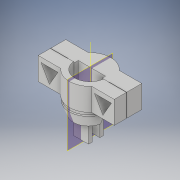
# Autodesk Inventor part: ECoG_holder_4p0
Saved by Autodesk Inventor 2017 (Build 210142000, 142)
## iProperties
Created: 2016-11-02
Part Number: ECoG_holder_4p0
Material: Generic
Document SubType Name: Modeling
Designer: Camilo
Density: 1 g/cm^3
Appearance: Default
Author: Camilo
Autodesk Inventor part; units mm, degrees
ref_plane "YZ Plane" through (0, 0, 0) normal (1, 0, 0) x (0, 1, 0)
ref_plane "XZ Plane" through (0, 0, 0) normal (0, 1, 0) x (-1, 0, 0)
ref_plane "XY Plane" through (0, 0, 0) normal (0, 0, 1) x (1, 0, 0)
sketch "Sketch1" plane through (0, 0, 0) normal (0, 0, 1) x (1, 0, 0)
  line L0 (0, 0) -> (0, -7.0002) construction
  line L1 (0, -7.0002) -> (0.78, -7.0002) construction
  line L2 (0.78, 0) -> (0.78, -7.0002) construction
  line L3 (0, 0) -> (0.78, 0) construction
  line L4 (0.39, -7.0002) -> (0.39, 0) construction
  circle A0 centre (0.39, -3.5001) radius 5.5
  dimension "d0" = 11
  constraints: 3 midpoint, 2 end point, 1 centre point
  measures "d0" diameter of A0
extrude "Extrusion1" add sketch "Sketch1" against normal blind 4.5 and the other way blind 1.5
shell "Shell1" thickness 1.5 removed faces 1 at (2.1701, -3.9389, -4.5)
sketch "Sketch2" plane through (0.39, -3.5001, 0) normal (0, 0, -1) x (-1, 0, 0)
  line L0 (0.39, 3.5001) -> (0.39, -3.5001) construction
  line L1 (0.39, -3.5001) -> (-0.39, -3.5001) construction
  line L2 (-0.39, 3.5001) -> (-0.39, -3.5001) construction
  line L3 (0.39, 3.5001) -> (-0.39, 3.5001) construction
  circle A0 centre (0, 0) radius 4 construction
  line L4 (0.515, -3.6251) -> (0.515, 3.6251)
  line L5 (0.515, 3.6251) -> (-0.515, 3.6251)
  line L6 (-0.515, 3.6251) -> (-0.515, -3.6251)
  line L7 (-0.515, -3.6251) -> (0.515, -3.6251)
  line L8 (-0.39, -3.6251) -> (-0.39, -3.9809)
  line L9 (-0.39, 3.6251) -> (-0.39, 3.9809)
  arc A1 (-0.39, -3.9809) -> (-0.39, 3.9809) centre (0, 0) ccw
  dimension "d6" = 0.125
  constraints: 12 end point, 4 point on circle, 4 point on line, 1 centre point, 1 vertical, 3 other
  measures "d6" distance between parallel lines of L0 L4
extrude "Extrusion2" add sketch "Sketch2" along normal up to surface (4.5 mm away) contours L4 L5 L9 A1 L8 L7
sketch "Sketch3" plane through (0.39, -3.5001, -4.5) normal (0, 0, -1) x (-1, 0, 0)
  arc A0 (-0.39, 3.9809) -> (-0.39, -3.9809) centre (0, 0) ccw construction
  line L0 (-0.39, 3.9809) -> (-0.39, 3.6251) construction
  line L1 (-0.39, 3.6251) -> (0.515, 3.6251) construction
  line L2 (0.515, 3.6251) -> (0.515, -3.6251) construction
  line L3 (0.515, -3.6251) -> (-0.39, -3.6251) construction
  line L4 (-0.39, -3.6251) -> (-0.39, -3.9809) construction
  circle A1 centre (0, 0) radius 5.5 construction
  circle A2 centre (0, 0) radius 5.5 projected
  line L5 (-0.39, -5.4862) -> (-0.39, 5.4862)
  point P0 (0.39, 3.5001)
  constraints: 4 point on circle, 2 end point, 1 point on line, 1 vertical
split body "Split1" sketch "Sketch3" result two bodies curves L5 first body at (4.651, -4.9471, -3)
sketch "Sketch11" plane through (0, 0, -4.5) normal (0, 0, -1) x (-1, 0, 0)
  line L0 (-0.78, 1.986) -> (-0.78, 0.125) construction
  line L1 (-0.78, 0.125) -> (0.125, 0.125) construction
  line L2 (0.125, 0.125) -> (0.125, -7.1252) construction
  line L3 (0.125, -7.1252) -> (-0.78, -7.1252) construction
  line L4 (-0.78, -7.1252) -> (-0.78, -8.9863) construction
  arc A0 (-0.78, -8.9863) -> (-0.78, 1.986) centre (-0.39, -3.5001) ccw construction
  arc A1 (-0.78, -8.9863) -> (-0.78, 1.986) centre (-0.39, -3.5001) ccw construction
  line L5 (-0.73, -13.6055) -> (3.27, -13.6055)
  line L6 (3.27, -13.6055) -> (3.27, -7.6055)
  line L7 (3.27, -7.6055) -> (-0.73, -7.6055)
  line L8 (-0.73, -7.6055) -> (-0.73, -13.6055)
  line L9 (-0.39, -3.5001) -> (5.11, -3.5001) construction
  line L10 (0.125, 0.125) -> (-0.78, 0.125) construction
  line L11 (-0.78, 0.125) -> (-0.78, 1.986) construction
  line L12 (-0.73, 6.6053) -> (3.27, 6.6053)
  line L13 (3.27, 6.6053) -> (3.27, 0.6053)
  line L14 (3.27, 0.6053) -> (-0.73, 0.6053)
  line L15 (-0.73, 0.6053) -> (-0.73, 6.6053)
  point P0 (0, 0)
  dimension "d38" = 0.05
  dimension "d39" = 4
  dimension "d40" = 6
  constraints: 22 end point, 4 symmetric about line, 3 point on circle, 2 parallel, 1 horizontal, 1 perpendicular
  measures "d38" distance between parallel lines of L8 L4
  measures "d39" distance of L5.start L5.end
  measures "d40" distance of L5.end L6.end
extrude "Extrusion10" add sketch "Sketch11" against normal up to surface (6 mm away) bodies 3
sketch "Sketch12" plane through (0, 0, -4.5) normal (0, 0, -1) x (-1, 0, 0)
  line L0 (-0.78, 1.986) -> (-0.78, 0.4808) construction
  arc A0 (-0.78, 1.986) -> (-5.89, -3.5001) centre (-0.39, -3.5001) ccw construction
  arc A1 (-5.89, -3.5001) -> (-0.78, -8.9863) centre (-0.39, -3.5001) ccw construction
  line L1 (-0.78, -7.4811) -> (-0.78, -8.9863) construction
  arc A2 (-0.78, 0.4808) -> (-0.78, -7.4811) centre (-0.39, -3.5001) ccw construction
  line L2 (-0.39, -3.5001) -> (-5.89, -3.5001) construction
  arc A3 (-0.78, 1.986) -> (-5.89, -3.5001) centre (-0.39, -3.5001) ccw projected
  line L3 (-0.83, 6.6053) -> (-4.05, 6.6053)
  line L4 (-4.05, 6.6053) -> (-4.05, 0.6053)
  line L5 (-4.05, 0.6053) -> (-0.83, 0.6053)
  line L6 (-0.83, 0.6053) -> (-0.83, 6.6053)
  line L7 (-0.73, 6.6053) -> (3.27, 6.6053) projected
  line L8 (-0.78, -8.9863) -> (-0.78, -7.4811) construction
  line L9 (-0.83, -13.6055) -> (-4.05, -13.6055)
  line L10 (-4.05, -13.6055) -> (-4.05, -7.6055)
  line L11 (-4.05, -7.6055) -> (-0.83, -7.6055)
  line L12 (-0.83, -7.6055) -> (-0.83, -13.6055)
  point P0 (0, 0)
  dimension "d43" = 0.05
  dimension "d44" = 6
  dimension "d46" = 0
  constraints: 20 end point, 4 symmetric about line, 2 horizontal, 2 parallel, 2 point on circle, 1 perpendicular
  measures "d43" distance between parallel lines of L6 L0
  measures "d44" distance of L3.end L4.end
  measures "d46" distance between parallel lines of L3 L7
extrude "Extrusion11" add sketch "Sketch12" against normal up to surface (6 mm away) bodies 2
sketch "Sketch13" plane through (0.73, 1.9894, -4.5) normal (1, 0, 0) x (0, 0, -1)
  line L0 (0, 0) -> (-6, 0) construction
  line L1 (0, 0) -> (0, 4.6159) construction
  line L2 (0, 4.6159) -> (-6, 4.6159) construction
  line L3 (-6, 4.6159) -> (-6, 0) construction
  line L4 (-6, -10.979) -> (0, -10.979) construction
  line L5 (-6, -10.979) -> (-6, -15.5949) construction
  line L6 (0, -15.5949) -> (-6, -15.5949) construction
  line L7 (0, -10.979) -> (0, -15.5949) construction
  line L8 (0, -1.8644) -> (0, -9.1146) construction
  line L9 (-4.5, -1.8644) -> (0, -1.8644) construction
  line L10 (-4.5, -9.1146) -> (-4.5, -1.8644) construction
  line L11 (-4.5, -9.1146) -> (0, -9.1146) construction
  line L12 (0, -10.9756) -> (-6, -10.9756) construction
  line L13 (0, -15.5949) -> (0, -9.5949) construction
  line L14 (-5.15, 1.6159) -> (-1.25, 3.8676)
  line L15 (-1.25, 3.8676) -> (-1.25, -0.6357)
  line L16 (-1.25, -0.6357) -> (-5.15, 1.6159)
  line L17 (-5.15, -12.5949) -> (-1.25, -10.3432)
  line L18 (-1.25, -10.3432) -> (-1.25, -14.8466)
  line L19 (-1.25, -14.8466) -> (-5.15, -12.5949)
  circle A0 centre (-2.55, 1.6159) radius 1.3
  point P0 (-4.5, -1.9894)
  point P1 (-2.55, -12.5949)
  dimension "d77" = 2.6
  dimension "d78" = 1.25
  dimension "d79" = 3
  dimension "d80" = 3
  constraints: 12 end point, 2 collinear, 2 vertical, 1 centre point, 1 coincident, 1 tangent, 14 other
  measures "d77" diameter of A0
  measures "d78" distance between parallel lines of L1 L15
  measures "d79" distance from line of point (-2.55, 1.616) L2
  measures "d80" distance from line of point (-2.55, -12.595) L6
extrude "Extrusion12" cut sketch "Sketch13" against normal blind 2.5 and the other way blind 0.2 bodies 3
sketch "Sketch14" plane through (0.83, 1.9823, -4.5) normal (-1, 0, 0) x (0, 0, 1)
  line L0 (1.25, 3.8747) -> (1.25, -0.6286) construction
  line L1 (5.15, 1.623) -> (1.25, 3.8747) construction
  line L2 (1.25, -0.6286) -> (5.15, 1.623) construction
  line L3 (5.15, -12.5878) -> (1.25, -10.3361) construction
  line L4 (1.25, -10.3361) -> (1.25, -14.8394) construction
  line L5 (1.25, -14.8394) -> (5.15, -12.5878) construction
  line L6 (1.25, 3.8747) -> (1.25, -0.6286)
  line L7 (1.25, -0.6286) -> (5.15, 1.623)
  line L8 (5.15, 1.623) -> (1.25, 3.8747)
  line L9 (1.25, -10.3361) -> (5.15, -12.5878)
  line L10 (5.15, -12.5878) -> (1.25, -14.8394)
  line L11 (1.25, -14.8394) -> (1.25, -10.3361)
  point P0 (4.5, -1.9823)
  dimension "d52" = 0
  constraints: 12 end point, 1 collinear, 4 other
  measures "d52" distance between parallel lines of L1 L8
extrude "Extrusion13" cut sketch "Sketch14" against normal through all bodies 2
sketch "Sketch15" plane through (0, 0, 1.5) normal (0, 0, 1) x (1, 0, 0)
  arc A0 (0.73, -8.9896) -> (0.78, -8.9863) centre (0.39, -3.5001) ccw construction
  line L0 (0.78, -8.9863) -> (0.78, 1.986) construction
  arc A1 (0.78, 1.986) -> (0.73, 1.9894) centre (0.39, -3.5001) ccw construction
  line L1 (0.73, 6.6053) -> (0.73, 1.9894) construction
  line L2 (-3.27, 6.6053) -> (0.73, 6.6053) construction
  line L3 (-3.27, 0.6053) -> (-3.27, 6.6053) construction
  arc A2 (-3.27, 0.6053) -> (-3.27, -7.6055) centre (0.39, -3.5001) ccw construction
  line L4 (-3.27, -13.6055) -> (-3.27, -7.6055) construction
  line L5 (0.73, -13.6055) -> (-3.27, -13.6055) construction
  line L6 (0.73, -8.9896) -> (0.73, -13.6055) construction
  line L7 (0.78, -1.0001) -> (-0.22, -1.0001)
  line L8 (-0.22, -1.0001) -> (-0.22, -6.0001)
  line L9 (-0.22, -6.0001) -> (0.78, -6.0001)
  line L10 (0.78, -6.0001) -> (0.78, -1.0001)
  line L11 (0.78, -0.0001) -> (-1.22, -0.0001)
  line L12 (-1.22, -0.0001) -> (-1.22, -7.0001)
  line L13 (-1.22, -7.0001) -> (0.78, -7.0001)
  line L14 (0.78, -7.0001) -> (0.78, -0.0001)
  line L15 (0.78, -8.9863) -> (0.78, 1.986) projected
  point P0 (0, 0)
  point P1 (0.78, -3.5001)
  point P2 (0.78, -3.5001)
  dimension "d55" = 5
  dimension "d56" = 1
  dimension "d57" = 1
  dimension "d58" = 1
  constraints: 16 end point, 4 midpoint, 4 parallel, 2 horizontal, 2 perpendicular
  measures "d55" distance of L7.end L8.end
  measures "d56" distance of L8.end L9.end
  measures "d57" distance between parallel lines of L12 L8
  measures "d58" distance between parallel lines of L9 L13
extrude "Extrusion14" add sketch "Sketch15" along normal blind 2 contours L7 L8 L9 L14 L13 L12 L11 bodies 3
sketch "Sketch16" plane through (0, 0, 1.5) normal (0, 0, 1) x (1, 0, 0)
  arc A0 (0.83, 1.9823) -> (0.78, 1.986) centre (0.39, -3.5001) ccw construction
  line L0 (0.78, -8.9863) -> (0.78, 1.986) construction
  arc A1 (0.78, -8.9863) -> (0.83, -8.9825) centre (0.39, -3.5001) ccw construction
  line L1 (0.83, -13.6055) -> (0.83, -8.9825) construction
  line L2 (4.05, -13.6055) -> (0.83, -13.6055) construction
  line L3 (4.05, -7.6055) -> (4.05, -13.6055) construction
  arc A2 (4.05, -7.6055) -> (4.05, 0.6053) centre (0.39, -3.5001) ccw construction
  line L4 (4.05, 6.6053) -> (4.05, 0.6053) construction
  line L5 (0.83, 6.6053) -> (4.05, 6.6053) construction
  line L6 (0.83, 1.9823) -> (0.83, 6.6053) construction
  line L7 (-0.22, -1.0001) -> (0.78, -1.0001) construction
  line L8 (0.78, -1.0001) -> (0.78, -0.0001) projected
  line L9 (0.78, -0.0001) -> (-1.22, -0.0001) construction
  line L10 (-1.22, -0.0001) -> (-1.22, -7.0001) construction
  line L11 (-1.22, -7.0001) -> (0.78, -7.0001) construction
  line L12 (0.78, -7.0001) -> (0.78, -6.0001) projected
  line L13 (0.78, -6.0001) -> (-0.22, -6.0001) construction
  line L14 (-0.22, -6.0001) -> (-0.22, -1.0001) construction
  line L15 (1.78, -1.0001) -> (0.78, -1.0001)
  line L16 (0.78, -0.0001) -> (2.78, -0.0001)
  line L17 (2.78, -0.0001) -> (2.78, -7.0001)
  line L18 (2.78, -7.0001) -> (0.78, -7.0001)
  line L19 (0.78, -6.0001) -> (1.78, -6.0001)
  line L20 (1.78, -6.0001) -> (1.78, -1.0001)
  point P0 (0, 0)
  point P1 (1.56, 0)
  point P2 (1.17, -3.5001)
  point P3 (1.17, -3.5001)
  point P4 (1.17, -3.5001)
  constraints: 12 end point, 8 symmetric about line
extrude "Extrusion15" add sketch "Sketch16" along normal blind 2 bodies 2
sketch "Sketch17" plane through (0.78, -7.1252, 0) normal (1, 0, 0) x (0, 0, -1)
  line L0 (-1.5, 9.1113) -> (4.5, 9.1113) projected
  line L1 (-1.5, 9.1113) -> (-1.5, 7.1113)
  line L2 (-1.5, 9.1113) -> (0.5, 9.1113) construction
  line L3 (-1.5, 7.1251) -> (-1.5, 9.1113) projected
  line L4 (-1.5, 7.1251) -> (-5.5, 7.1251)
  line L5 (-5.5, 7.1251) -> (-5.5, 7.6251)
  line L6 (-5.5, 7.6251) -> (-1.5, 9.1113)
  line L7 (-7.5, 3.6251) -> (6.5, 3.6251) projected
  line L8 (-2, 8.9255) -> (-1.5, 8.9255) construction
  line L9 (-1.5, 8.9255) -> (-1.5, 8.6255)
  line L10 (-1.5, 8.6255) -> (-2, 8.6255)
  line L11 (-2, 8.6255) -> (-2, 8.9255)
  point P0 (0, 7.1252)
  dimension "d63" = 2
  dimension "d64" = 90
  dimension "d65" = 4
  dimension "d66" = 0.5
  dimension "d69" = 0.5
  dimension "d70" = 0.3
  constraints: 18 end point, 3 horizontal, 3 perpendicular, 2 parallel, 2 point on line, 1 vertical
  measures "d63" distance of L0.start L1.end
  measures "d64" angle of L1 L2
  measures "d65" distance of L3.start L4.end
  measures "d66" distance of L4.end L5.end
  measures "d69" distance of L9.end L10.end
  measures "d70" distance of L10.end L8.start
revolve "Revolution1" add sketch "Sketch17" angle 180 about axis through (0.78, -3.5001, 0) along (0, 0, 1) bodies 3
sketch "Sketch18" plane through (0.78, -7.1252, 0) normal (-1, 0, 0) x (0, 0, 1)
  line L0 (-2.1546, -1.861) -> (1.5, -1.861) construction
  line L1 (-4.5, 0) -> (-4.5, -1.861) construction
  line L2 (0, 0) -> (-4.5, 0) construction
  line L3 (0, 7.2502) -> (0, 0) construction
  line L4 (0, 7.2502) -> (-4.5, 7.2502) construction
  line L5 (-4.5, 9.1113) -> (-4.5, 7.2502) construction
  line L6 (1.5, 9.1113) -> (-2.1546, 9.1113) construction
  line L7 (5.5, 7.6251) -> (1.5, 9.1113) construction
  line L8 (5.5, 7.1251) -> (5.5, 7.6251) construction
  line L9 (3.5, 7.1251) -> (5.5, 7.1251) construction
  line L10 (3.5, 6.1251) -> (3.5, 7.1251) construction
  line L11 (3.5, 6.1251) -> (1.5, 6.1251) construction
  line L12 (1.5, 1.1251) -> (1.5, 6.1251) construction
  line L13 (1.5, 1.1251) -> (3.5, 1.1251) construction
  line L14 (3.5, 0.1251) -> (3.5, 1.1251) construction
  line L15 (3.5, 0.1251) -> (5.5, 0.1251) construction
  line L16 (5.5, 0.1251) -> (5.5, -0.3749) construction
  line L17 (5.5, -0.3749) -> (1.5, -1.861) construction
  line L18 (5.5, 7.6251) -> (1.5, 9.1113) projected
  line L19 (1.5, 7.1251) -> (3.5, 7.1251) projected
  line L20 (1.5, 9.1113) -> (1.5, 7.1251)
  line L21 (1.5, 7.1251) -> (5.5, 7.1251)
  line L22 (1.5, 9.1113) -> (1.5, -1.861) projected
  line L23 (5.5, 7.6251) -> (1.5, 9.1113)
  line L24 (5.5, 7.1251) -> (5.5, 7.6251) projected
  line L25 (5.5, 7.1251) -> (5.5, 7.6251)
  line L26 (7.5, 3.6251) -> (-6.5, 3.6251) projected
  line L27 (-3.25, 8.4789) -> (-2.1546, 9.1113) projected
  line L28 (-2.1546, -1.861) -> (-3.25, -1.2286) projected
  line L29 (-3.25, -1.2286) -> (-3.25, -1.861) projected
  line L30 (-4.5, -1.861) -> (-3.25, -1.861) projected
  line L31 (-3.25, 9.1113) -> (-4.5, 9.1113) projected
  line L32 (-3.25, 9.1113) -> (-3.25, 8.4789) projected
  point P0 (0, 7.1252)
  constraints: 8 end point, 2 collinear, 2 perpendicular
revolve "Revolution2" add sketch "Sketch18" angle 180 about axis through (0.78, -3.5001, 0) along (0, 0, -1) bodies 2
sketch "Sketch19" plane through (0.78, -7.1252, 0) normal (1, 0, 0) x (0, 0, -1)
  line L0 (2.1546, -1.861) -> (-1.5, -1.861) construction
  line L1 (4.5, 0) -> (4.5, -1.861) construction
  line L2 (0, 0) -> (4.5, 0) construction
  line L3 (0, 7.2502) -> (0, 0) construction
  line L4 (0, 7.2502) -> (4.5, 7.2502) construction
  line L5 (4.5, 9.1113) -> (4.5, 7.2502) construction
  line L6 (-1.5, 9.1113) -> (2.1546, 9.1113) construction
  line L7 (-5.5, 7.6251) -> (-1.5, 9.1113) construction
  line L8 (-5.5, 7.1251) -> (-5.5, 7.6251) construction
  line L9 (-3.5, 7.1251) -> (-5.5, 7.1251) construction
  line L10 (-3.5, 6.1251) -> (-3.5, 7.1251) construction
  line L11 (-3.5, 6.1251) -> (-1.5, 6.1251) construction
  line L12 (-1.5, 1.1251) -> (-1.5, 6.1251) construction
  line L13 (-1.5, 1.1251) -> (-3.5, 1.1251) construction
  line L14 (-3.5, 0.1251) -> (-3.5, 1.1251) construction
  line L15 (-3.5, 0.1251) -> (-5.5, 0.1251) construction
  line L16 (-5.5, 0.1251) -> (-5.5, -0.3749) construction
  line L17 (-5.5, -0.3749) -> (-1.5, -1.861) construction
  line L18 (-1.5, 9.1113) -> (-2.5, 8.7397)
  line L19 (-2.5, 8.7397) -> (-1.5, 8.7397)
  line L20 (-1.5, 8.7397) -> (-1.5, 9.1113)
  line L21 (-2.5, 8.7397) -> (-1.5, 8.7397)
  line L22 (-1.5, 8.7397) -> (-1.5, 8.5276)
  line L23 (-1.5, 8.5276) -> (-2.2879, 8.5276)
  line L24 (-2.2879, 8.5276) -> (-2.5, 8.7397)
  line L25 (-7.5, 3.6251) -> (6.5, 3.6251) projected
  line L26 (-1.5, 7.7305) -> (-1.5, 13.7305) projected
  line L27 (3.25, 8.4789) -> (2.1546, 9.1113) projected
  line L28 (2.1546, -1.861) -> (3.25, -1.2286) projected
  line L29 (3.25, -1.2286) -> (3.25, -1.861) projected
  line L30 (4.5, -1.861) -> (3.25, -1.861) projected
  line L31 (3.25, 9.1113) -> (4.5, 9.1113) projected
  line L32 (3.25, 9.1113) -> (3.25, 8.4789) projected
  point P0 (0, 7.1252)
  dimension "d71" = 1
  dimension "d72" = 0.3
  dimension "d75" = 135
  constraints: 14 end point, 2 horizontal, 2 perpendicular, 1 collinear, 1 parallel, 1 point on line
  measures "d71" distance of L18.end L19.end
  measures "d72" distance of L23.end L18.end
  measures "d75" angle of L24 L23
revolve "Revolution3" cut sketch "Sketch19" angle 180 about axis through (0.78, -3.5001, 0) along (0, 0, 1) bodies 3
sketch "Sketch21" plane through (0.78, -7.1252, 0) normal (-1, 0, 0) x (0, 0, 1)
  line L0 (1.5, 8.5276) -> (2.2879, 8.5276) projected
  line L1 (2.2879, 8.5276) -> (2.5, 8.7397) projected
  line L2 (5.5, 7.6251) -> (1.5, 9.1113) projected
  line L3 (1.5, 7.7305) -> (1.5, 13.7305) projected
  line L4 (7.5, 3.6251) -> (-6.5, 3.6251) projected
  point P0 (0, 7.1252)
revolve "Revolution5" cut sketch "Sketch21" angle 180 about axis through (0.78, -3.5001, 0) along (0, 0, -1) bodies 2
sketch "Sketch22" plane through (0, 0, 1.5) normal (0, 0, 1) x (1, 0, 0)
  arc A0 (2.78, -6.3724) -> (2.78, -0.6278) centre (0.78, -3.5001) ccw projected
  line L0 (2.78, -0.6278) -> (2.78, -6.3724) projected
  point P0 (0, 0)
extrude "Extrusion16" add sketch "Sketch22" along normal up to surface (2 mm away) bodies 2
sketch "Sketch23" plane through (0, 0, 1.5) normal (0, 0, 1) x (1, 0, 0)
  arc A0 (-1.22, -0.6278) -> (-1.22, -6.3724) centre (0.78, -3.5001) ccw projected
  line L0 (-1.22, -6.3724) -> (-1.22, -0.6278) projected
  point P0 (0, 0)
extrude "Extrusion17" add sketch "Sketch23" along normal up to surface (2 mm away) bodies 3
sketch "Sketch24" plane through (0, 0, 3.5) normal (0, 0, 1) x (1, 0, 0)
  line L0 (1.78, -1.0001) -> (1.78, -6.0001) construction
  line L1 (0.78, -1.5001) -> (0.78, -5.5001)
  line L2 (0.78, -5.5001) -> (2.78, -5.5001)
  line L3 (2.78, -5.5001) -> (2.78, -1.5001)
  line L4 (2.78, -1.5001) -> (0.78, -1.5001)
  line L5 (1.78, -6.0001) -> (1.78, -1.0001) projected
  line L6 (0.78, -1.5001) -> (2.78, -5.5001) construction
  line L7 (0.78, -5.5001) -> (2.78, -1.5001) construction
  line L8 (1.78, -5.5001) -> (1.78, -1.5001)
  point P0 (0, 0)
  point P1 (1.78, -3.5001)
  dimension "d87" = 4
  dimension "d88" = 2
  constraints: 14 end point, 5 midpoint, 2 parallel, 2 point on line, 1 perpendicular
  measures "d87" distance of L1.start L1.end
  measures "d88" distance of L2.end L1.end
extrude "Extrusion18" add sketch "Sketch24" along normal blind 7 contours L4 L3 L2 L5 bodies 2
sketch "Sketch25" plane through (0, 0, 3.5) normal (0, 0, 1) x (1, 0, 0)
  line L0 (-0.22, -6.0001) -> (-0.22, -1.0001) projected
  line L1 (1.78, -5.5001) -> (2.78, -5.5001) projected
  line L2 (0.78, -1.5001) -> (0.78, -5.5001)
  line L3 (0.78, -5.5001) -> (-1.22, -5.5001)
  line L4 (-1.22, -5.5001) -> (-1.22, -1.5001)
  line L5 (-1.22, -1.5001) -> (0.78, -1.5001)
  line L6 (0.78, -1.5001) -> (-1.22, -5.5001) construction
  line L7 (0.78, -5.5001) -> (-1.22, -1.5001) construction
  line L8 (2.78, -5.5001) -> (2.78, -1.5001) projected
  line L9 (-0.22, -3.5001) -> (-1.22, -3.5001) construction
  line L10 (-0.22, -5.5001) -> (-0.22, -1.5001)
  point P0 (0, 0)
  constraints: 16 end point, 6 midpoint, 4 parallel, 1 perpendicular, 1 point on line
extrude "Extrusion19" add sketch "Sketch25" along normal up to surface (7 mm away) contours L3 L4 L5 L0 bodies 3
ref_plane "Work Plane1" through (1.78, -3.5001, 3.5) normal (0, -1, 0) x (1, 0, 0)
sketch "Sketch26" plane through (1.78, -3.5001, 3.5) normal (0, -1, 0) x (1, 0, 0)
  line L0 (-1, 2) -> (3, 2) projected
  line L1 (-1, 0) -> (2.5, 0) projected
  line L2 (-1, -1) -> (-1, -1) projected
  line L3 (-1, 2) -> (-1, -1) projected
  line L4 (-1, 2) -> (-1, 2) projected
  line L5 (-1, -1) -> (-1, 2) projected
  line L6 (-1, 0) -> (-0.25, 0)
  line L7 (-0.25, 0) -> (-0.25, 2)
  line L8 (-0.25, 2) -> (-1, 2)
  line L9 (-1, 2) -> (-1, 0)
  point P0 (-1.78, -3.5)
  dimension "d93" = 0.75
  constraints: 8 end point, 2 parallel, 1 horizontal, 1 perpendicular, 1 point on line
  measures "d93" distance between parallel lines of L3 L7
extrude "Extrusion20" cut sketch "Sketch26" along normal through all both and the other way through all bodies 2
ref_plane "Work Plane2" through (-1.22, -3.5001, 3.5) normal (0, 1, 0) x (1, 0, 0)
sketch "Sketch27" plane through (-1.22, -3.5001, 3.5) normal (0, 1, 0) x (1, 0, 0)
  line L0 (-2, -2) -> (2, -2) projected
  line L1 (2, 0) -> (-1.5, 0) projected
  line L2 (2, 1) -> (2, 1) projected
  line L3 (2, -2) -> (2, 1) projected
  line L4 (2, -2) -> (2, -2) projected
  line L5 (2, -2) -> (2, 1) projected
  line L6 (2, 0) -> (1.25, 0)
  line L7 (1.25, 0) -> (1.25, -2)
  line L8 (1.25, -2) -> (2, -2)
  line L9 (2, -2) -> (2, 0)
  point P0 (1.22, 3.5)
  dimension "d96" = 0.75
  constraints: 8 end point, 2 parallel, 1 horizontal, 1 perpendicular, 1 point on line
  measures "d96" distance between parallel lines of L3 L7
extrude "Extrusion21" cut sketch "Sketch27" along normal through all both and the other way through all bodies 3
body "Solid2"
body "Solid3"
